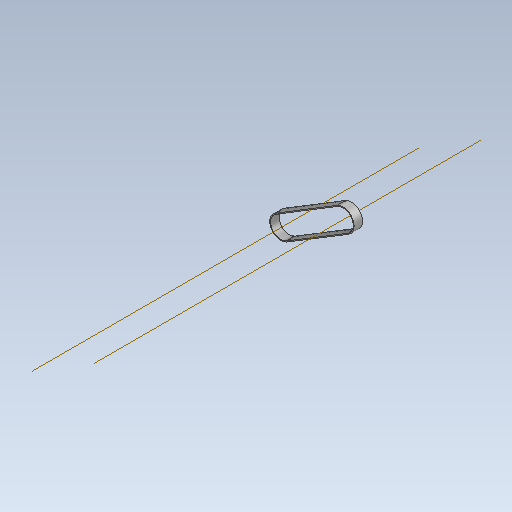
# Autodesk Inventor part: Synchronous Belt
Saved by Autodesk Inventor 2020 (Build 240168000, 168)
## iProperties
Created: 2022-07-18
Part Number: Synchronous Belt
Material: Rubber
Document SubType Name: Modeling
Designer: karimi2
Density: 1 g/cm^3
Appearance: Rubber - Black - Version 1.1
CustomPartVersion: 1
Author: karimi2
Autodesk Inventor part; units mm, degrees
ref_plane "YZ Plane" through (0, 0, 0) normal (1, 0, 0) x (0, 1, 0)
ref_plane "XZ Plane" through (0, 0, 0) normal (0, 1, 0) x (-1, 0, 0)
ref_plane "XY Plane" through (0, 0, 0) normal (0, 0, 1) x (1, 0, 0)
sketch "Sketch Path" plane through (0, 0, 0) normal (0, 0, 1) x (1, 0, 0)
  arc A0 (-114.429962, -59.867024) -> (-106.009882, -73.671941) centre (-110.219922, -66.769483) ccw
  arc A1 (-59.114981, -45.069176) -> (-67.535061, -31.264258) centre (-63.325021, -38.166717) ccw
  line L0 (-59.114981, -45.069176) -> (-106.009882, -73.671941)
  line L1 (-114.429962, -59.867024) -> (-67.535061, -31.264258)
  constraints: 4 end point, 4 point on circle, 2 centre point
ref_plane "Cross Section Plane" through (-106.009882, -73.671941, 0) normal (0.8537289, 0.5207177, 0) x (0, 0, 1)
ref_plane "Work Plane2" through (-110.219922, -66.769483, 0) normal (-1, 0, 0) x (0, 0, 1)
ref_plane "Work Plane3" through (-63.325021, -38.166717, 0) normal (-0.8723751, -0.4888371, 0) x (0, 0, 1)
sketch "Cross Section" plane through (-106.009882, -73.671941, 0) normal (0.8537289, 0.5207177, 0) x (0, 0, 1)
  line L0 (-3.175, 0.381) -> (3.175, 0.381)
  line L1 (3.175, 0.381) -> (3.175, -0.254)
  line L2 (3.175, -0.254) -> (-3.175, -0.254)
  line L3 (-3.175, -0.254) -> (-3.175, 0.381)
  line L4 (-3.175, 0) -> (3.175, 0) construction
  point P0 (0, 0)
  point P1 (0, 0)
  dimension "d0" = 6.35
  dimension "d4" = 0.254
  dimension "d5" = 0.381
  constraints: 10 end point, 2 parallel, 2 point on line, 1 coincident, 1 horizontal, 1 midpoint, 1 perpendicular, 1 other
  measures "d0" distance between parallel lines of L1 L3
  measures "d4" distance between parallel lines of L2 L4
  measures "d5" distance between parallel lines of L4 L0
sweep "Belt" add profiles "Cross Section" path "Sketch Path" path curves L1 A1 L0 A0
equation "\"d0\" = da_B"
equation "\"d4\" = da_a"
equation "\"d5\" = da_a2"
equation "\"da_B\" = 6.35"
equation "\"da_pb\" = 2.032"
equation "\"da_L\" = 160.659"
equation "\"da_a\" = 0.254"
equation "\"da_S\" = 1.143"
equation "\"da_Beta\" = 20deg"
equation "\"da_Ht\" = 0.508"
equation "\"da_H\" = 1.143"
equation "\"da_a2\" = 0.381"
body "Solid1"
